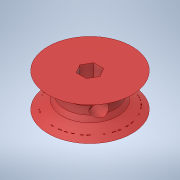
# Autodesk Inventor part: hexSpoolForArmV01
Saved by Autodesk Inventor 2022.2 (Build 262287010, 287A)
## iProperties
Created: 2019-02-24
Part Number: hexSpoolForArmV01
Material: PC/ABS Plastic
Document SubType Name: Modeling
Designer: steele
Density: 0.357273 g/cm^3
Appearance: Smooth - Red
holeForString: 0.200 in
stringDiameter: 0.120 in
clearanceForString: 0.080 in
clearanceForHexShaft: 0.020 in
spoolInteriorDiameter: 1.500 in
spoolInteriroRadius: 0.750 in
spoolExteriorDiameter: 2.500 in
spoolExteriorRadius: 1.250 in
hexHoleChamfer: 0.063 in
stringHoleCenterFromHexShaft: 0.360 in
textCircleDiameter: 1.875 in
textHeight: 0.180 in
textDepth: 0.050 in
Author: steele
Autodesk Inventor part; units mm, degrees
(part 1 of 2)
ref_plane "XZ Plane" through (0, 0, 0) normal (0, 1, 0) x (-1, 0, 0)
ref_plane "XY Plane" through (0, 0, 0) normal (0, 0, 1) x (1, 0, 0)
sketch "Sketch15" plane through (0, 0, 0) normal (0, 0, 1) x (1, 0, 0)
  line L0 (31.75, 0) -> (31.75, 50.8) construction
  line L1 (12.065, 0) -> (31.75, 0)
  line L2 (19.05, 0) -> (19.05, 50.8) construction
  line L3 (0, 50.8) -> (0, 0)
  line L4 (19.05, 12.7) -> (31.75, 12.7) construction
  line L5 (31.75, 0) -> (19.05, 7.3323)
  line L6 (31.75, 25.4) -> (19.05, 18.0677)
  line L7 (19.05, 18.0677) -> (31.75, 18.0677) construction
  line L8 (19.05, 18.0677) -> (19.05, 7.3323)
  line L9 (31.75, 25.4) -> (19.05, 32.7323)
  line L10 (19.05, 32.7323) -> (19.05, 43.4677)
  line L11 (19.05, 43.4677) -> (31.75, 50.8)
  line L12 (31.75, 25.4) -> (19.05, 25.4) construction
  line L13 (19.05, 43.4677) -> (31.75, 43.4677) construction
  line L14 (12.065, 0) -> (0, 0)
  line L15 (31.75, 50.8) -> (0, 50.8)
  dimension "d86" = 50.8
  dimension "d89" = 25.4
  dimension "centerLineForSpool" = 12.7
  dimension "d93" = 30
  dimension "d94" = 30
  dimension "d95" = 30
  dimension "d96" = 30
  dimension "d156" = 31.75
  dimension "d158" = 31.75
  constraints: 32 end point, 9 point on line, 3 horizontal, 2 midpoint, 2 perpendicular, 1 collinear, 1 vertical
  measures "d86" distance of L0.start L0.end
  measures "d89" distance from line of L6.start L1
  measures "centerLineForSpool" distance from line of L4.start L1
  measures "d93" angle of L5 L1
  measures "d94" angle of L6 L7
  measures "d95" angle of L9 L12
  measures "d96" angle of L11 L13
  measures "d156" distance from line of L0.end L3
  measures "d158" distance from line of L0.start L3
revolve "Revolution2" add sketch "Sketch15" angle 360 about axis through (0, 50.8, 0) along (0, -1, 0)
sketch "Sketch16" plane through (0, 0, 0) normal (0, -1, 0) x (1, 0, 0)
  line L0 (-7.6256, 0) -> (-3.8128, 6.604)
  line L1 (-3.8128, 6.604) -> (3.8128, 6.604)
  line L2 (3.8128, 6.604) -> (7.6256, 0)
  line L3 (7.6256, 0) -> (3.8128, -6.604)
  line L4 (3.8128, -6.604) -> (-3.8128, -6.604)
  line L5 (-3.8128, -6.604) -> (-7.6256, 0)
  point P0 (0, 0)
  point P1 (0, 0)
  dimension "d103" = 13.208
  constraints: 12 end point, 1 coincident, 1 horizontal, 13 other
  measures "d103" distance between parallel lines of L1 L4
extrude "Extrusion11" cut sketch "Sketch16" against normal through all
sketch "Sketch17" plane through (0, 0, 0) normal (1, 0, 0) x (0, 1, 0)
  circle A0 centre (38.1, 9.144) radius 2.54
  circle A1 centre (12.7, 9.144) radius 2.54
  line L0 (0, 31.75) -> (0, -31.75) projected
  line L1 (50.8, 31.75) -> (50.8, -31.75) projected
  line L2 (0, 6.604) -> (50.8, 6.604) projected
  point P0 (0, 0)
  point P1 (50.8, -31.75)
  point P2 (69.85, 6.858)
  point P3 (72.39, 6.858)
  point P4 (50.8, 6.604)
  dimension "d110" = 12.7
  dimension "d111" = 12.7
  dimension "d112" = 5.08
  constraints: 2 centre point, 1 equal radius, 4 other
  measures "d110" distance from line of A1.centre L0
  measures "d112" diameter of A0
extrude "Extrusion13" cut sketch "Sketch17" along normal through all both and the other way through all
ref_plane "Work Plane4" through (-19.05, 0, 0) normal (1, 0, 0) x (0, 1, 0)
sketch "Sketch22" plane through (-19.05, 0, 0) normal (1, 0, 0) x (0, 1, 0)
  spline S0 degree 8 poles (40.64, 9.144) (40.64, 9.42) (40.6057, 9.6896) (40.54, 9.9488) (40.4456, 10.1945) (40.3253, 10.4241) (40.1822, 10.6353) (40.019, 10.8263) (39.6643, 11.1594) (39.4723, 11.3044) (39.2651, 11.4282) (39.0456, 11.5293) (38.8165, 11.6061) (38.5806, 11.6579) (38.3408, 11.684) (37.8188, 11.684) (37.5395, 11.6484) (37.2666, 11.5781) (37.0042, 11.4743) (36.7566, 11.3384) (36.5278, 11.1726) (36.322, 10.9796) (35.9648, 10.5477) (35.8095, 10.305) (35.6834, 10.0377) (35.5915, 9.75) (35.5382, 9.4472) (35.5271, 9.1354) (35.5605, 8.8213) (35.7533, 8.0702) (35.9537, 7.6667) (36.2256, 7.316) (36.5542, 7.0287) (36.9234, 6.8124) (37.3159, 6.6712) (37.7136, 6.604) (38.3775, 6.604) (38.6564, 6.6386) (38.9325, 6.7085) (39.2015, 6.8141) (39.4588, 6.9552) (39.6993, 7.1318) (39.9175, 7.3429) (40.2331, 7.7498) (40.3461, 7.9265) (40.4431, 8.1154) (40.522, 8.3139) (40.5815, 8.5192) (40.6208, 8.7281) (40.64, 8.9374) (40.64, 9.144) knots 0 0 0 0 0 0 0 0 0 0.12897 0.12897 0.12897 0.12897 0.12897 0.12897 0.12897 0.253758 0.253758 0.253758 0.253758 0.253758 0.253758 0.253758 0.399502 0.399502 0.399502 0.399502 0.399502 0.399502 0.399502 0.544455 0.544455 0.544455 0.544455 0.544455 0.544455 0.544455 0.751871 0.751871 0.751871 0.751871 0.751871 0.751871 0.751871 0.90085 0.90085 0.90085 0.90085 0.90085 0.90085 0.90085 1 1 1 1 1 1 1 1 1 projected
  circle A0 centre (38.1, 9.144) radius 4.7625
  circle A1 centre (38.1, 9.144) radius 2.54 construction
  line L0 (38.1, 6.604) -> (12.7, 6.604) construction
  line L1 (50.8, 31.75) -> (50.8, -31.75) construction
  point P0 (0, 0)
  point P1 (69.85, 6.858)
  point P2 (50.8, -31.75)
  point P3 (72.39, 6.858)
  point P4 (12.7, 6.604)
  dimension "d121" = 12.7
  dimension "d122" = 5.08
  dimension "d125" = 9.525
  constraints: 2 centre point, 1 concentric, 1 vertical alignment, 3 other
  measures "d122" diameter of A1
  measures "d125" diameter of A0
extrude "Extrusion16" cut sketch "Sketch22" along normal blind 11.1125
ref_plane "Work Plane5" through (19.05, 0, 0) normal (1, 0, 0) x (0, 1, 0)
sketch "Sketch23" plane through (19.05, 0, 0) normal (1, 0, 0) x (0, 1, 0)
  line L0 (12.7, 6.604) -> (38.1, 6.604) projected
  circle A0 centre (12.7, 9.144) radius 2.54 construction
  line L1 (0, 31.75) -> (0, -31.75) projected
  circle A1 centre (12.7, 9.144) radius 4.7625
  point P0 (0, 0)
  dimension "d127" = 5.08
  dimension "d128" = 12.7
  dimension "d129" = 9.525
  constraints: 2 centre point, 1 coincident, 1 tangent
  measures "d127" diameter of A0
  measures "d128" distance from line of A0.centre L1
  measures "d129" diameter of A1
extrude "Extrusion17" cut sketch "Sketch23" against normal blind 11.1125
chamfer "Chamfer12" distance 2.3813 angle 45 4 edges at (-19.05, 43.4677, 0) (-19.05, 32.7323, 0) (-19.05, 18.0677, 0) (-19.05, 7.3323, 0)
ref_plane "Work Plane6" through (0, 25.4, 0) normal (0, -1, 0) x (1, 0, 0)
sketch "Sketch26" plane through (0, 0, 0) normal (0, -1, 0) x (1, 0, 0)
  circle A0 centre (0, 0) radius 23.8125 construction
  spline S0 degree 2 poles (-24.7852, 3.5176) (-24.5019, 3.4962) (-24.0902, 3.2484) (-23.9621, 3.0591) knots 0 0 0 1 2 2 2
  spline S1 degree 2 poles (-23.9621, 3.0591) (-23.809, 2.8308) (-23.706, 2.3091) (-23.7359, 1.9119) knots 0 0 0 1 2 2 2
  line L0 (-23.7359, 1.9119) -> (-23.8505, 0.3941)
  line L1 (-23.8505, 0.3941) -> (-27.6497, 0.6808)
  line L2 (-27.6497, 0.6808) -> (-27.5486, 2.02)
  spline S2 degree 2 poles (-27.5486, 2.02) (-27.517, 2.4388) (-27.4198, 2.8649) (-27.3041, 3.045) knots 0 0 0 1 2 2 2
  spline S3 degree 2 poles (-27.3041, 3.045) (-27.1807, 3.2432) (-26.7962, 3.4154) (-26.556, 3.3973) knots 0 0 0 1 2 2 2
  spline S4 degree 2 poles (-26.556, 3.3973) (-26.2789, 3.3764) (-25.8657, 3.0665) (-25.7827, 2.8126) knots 0 0 0 1 2 2 2
  line L3 (-25.7827, 2.8126) -> (-25.7643, 2.8112)
  spline S5 degree 2 poles (-25.7643, 2.8112) (-25.6637, 3.1597) (-25.1731, 3.5468) (-24.7852, 3.5176) knots 0 0 0 1 2 2 2
  spline S6 degree 2 poles (-24.8749, 2.5335) (-25.0535, 2.547) (-25.2643, 2.4205) (-25.3273, 2.2828) knots 0 0 0 1 2 2 2
  spline S7 degree 2 poles (-25.3273, 2.2828) (-25.3677, 2.1992) (-25.3968, 1.8948) (-25.4159, 1.6424) knots 0 0 0 1 2 2 2
  line L4 (-25.4159, 1.6424) -> (-25.4291, 1.4669)
  line L5 (-25.4291, 1.4669) -> (-24.4716, 1.3946)
  line L6 (-24.4716, 1.3946) -> (-24.4677, 1.447)
  spline S8 degree 2 poles (-24.4677, 1.447) (-24.4398, 1.8164) (-24.4277, 2.1004) (-24.4812, 2.253) knots 0 0 0 1 2 2 2
  spline S9 degree 2 poles (-24.4812, 2.253) (-24.5299, 2.3867) (-24.7364, 2.5231) (-24.8749, 2.5335) knots 0 0 0 1 2 2 2
  spline S10 degree 2 poles (-26.4414, 2.4133) (-26.5338, 2.4203) (-26.7349, 2.3395) (-26.7855, 2.2442) knots 0 0 0 1 2 2 2
  spline S11 degree 2 poles (-26.7855, 2.2442) (-26.8355, 2.1551) (-26.8612, 1.897) (-26.8805, 1.6414) knots 0 0 0 1 2 2 2
  line L7 (-26.8805, 1.6414) -> (-26.8854, 1.5768)
  line L8 (-26.8854, 1.5768) -> (-26.0787, 1.5159)
  line L9 (-26.0787, 1.5159) -> (-26.0697, 1.636)
  spline S12 degree 2 poles (-26.0697, 1.636) (-26.0513, 1.8792) (-26.0457, 2.0769) (-26.0871, 2.1853) knots 0 0 0 1 2 2 2
  spline S13 degree 2 poles (-26.0871, 2.1853) (-26.1339, 2.3034) (-26.3152, 2.4038) (-26.4414, 2.4133) knots 0 0 0 1 2 2 2
  spline S14 degree 2 poles (-24.3269, 6.9191) (-23.6337, 6.7652) (-23.0058, 5.832) (-23.159, 5.1418) knots 0 0 0 1 2 2 2
  spline S15 degree 2 poles (-23.159, 5.1418) (-23.3116, 4.4545) (-24.2766, 3.8686) (-24.9698, 4.0224) knots 0 0 0 1 2 2 2
  spline S16 degree 2 poles (-24.9698, 4.0224) (-25.6691, 4.1776) (-26.2926, 5.1162) (-26.1401, 5.8034) knots 0 0 0 1 2 2 2
  spline S17 degree 2 poles (-26.1401, 5.8034) (-25.9875, 6.4906) (-25.0232, 7.0736) (-24.3269, 6.9191) knots 0 0 0 1 2 2 2
  spline S18 degree 2 poles (-24.5196, 6.0225) (-24.7698, 6.078) (-25.1224, 6.0709) (-25.2379, 6.0207) knots 0 0 0 1 2 2 2
  spline S19 degree 2 poles (-25.2379, 6.0207) (-25.3608, 5.9657) (-25.4857, 5.7878) (-25.5131, 5.6643) knots 0 0 0 1 2 2 2
  spline S20 degree 2 poles (-25.5131, 5.6643) (-25.5399, 5.5437) (-25.5097, 5.3377) (-25.4246, 5.2366) knots 0 0 0 1 2 2 2
  spline S21 degree 2 poles (-25.4246, 5.2366) (-25.3449, 5.1399) (-25.0243, 4.9738) (-24.7651, 4.9163) knots 0 0 0 1 2 2 2
  spline S22 degree 2 poles (-24.7651, 4.9163) (-24.5089, 4.8594) (-24.1737, 4.8736) (-24.0618, 4.9215) knots 0 0 0 1 2 2 2
  spline S23 degree 2 poles (-24.0618, 4.9215) (-23.95, 4.9694) (-23.8127, 5.1604) (-23.7846, 5.287) knots 0 0 0 1 2 2 2
  spline S24 degree 2 poles (-23.7846, 5.287) (-23.7612, 5.3924) (-23.8035, 5.6295) (-23.8792, 5.7159) knots 0 0 0 1 2 2 2
  spline S25 degree 2 poles (-23.8792, 5.7159) (-23.968, 5.8147) (-24.2543, 5.9636) (-24.5196, 6.0225) knots 0 0 0 1 2 2 2
  spline S26 degree 2 poles (-22.3455, 8.0742) (-22.5236, 7.5576) (-23.1127, 7.2315) (-23.5973, 7.3985) knots 0 0 0 1 2 2 2
  line L10 (-23.5973, 7.3985) -> (-24.8671, 7.8361)
  line L11 (-24.8671, 7.8361) -> (-24.9787, 7.5121)
  line L12 (-24.9787, 7.5121) -> (-25.5684, 7.7153)
  line L13 (-25.5684, 7.7153) -> (-25.4567, 8.0393)
  line L14 (-25.4567, 8.0393) -> (-26.2332, 8.3069)
  line L15 (-26.2332, 8.3069) -> (-25.9415, 9.1534)
  line L16 (-25.9415, 9.1534) -> (-25.165, 8.8858)
  line L17 (-25.165, 8.8858) -> (-24.8834, 9.7031)
  line L18 (-24.8834, 9.7031) -> (-24.2937, 9.4999)
  line L19 (-24.2937, 9.4999) -> (-24.5754, 8.6826)
  line L20 (-24.5754, 8.6826) -> (-23.6092, 8.3497)
  spline S27 degree 2 poles (-23.6092, 8.3497) (-23.4661, 8.3004) (-23.251, 8.2328) (-23.1543, 8.2386) knots 0 0 0 1 2 2 2
  spline S28 degree 2 poles (-23.1543, 8.2386) (-23.0576, 8.2445) (-22.899, 8.3825) (-22.8426, 8.546) knots 0 0 0 1 2 2 2
  spline S29 degree 2 poles (-22.8426, 8.546) (-22.8185, 8.616) (-22.8014, 8.8551) (-22.8097, 8.9069) knots 0 0 0 1 2 2 2
  line L21 (-22.8097, 8.9069) -> (-22.7846, 8.9799)
  line L22 (-22.7846, 8.9799) -> (-22.1891, 8.7747)
  spline S30 degree 2 poles (-22.1891, 8.7747) (-22.2013, 8.6254) (-22.2671, 8.3019) (-22.3455, 8.0742) knots 0 0 0 1 2 2 2
  spline S31 degree 2 poles (-21.5159, 10.0789) (-21.7403, 9.5806) (-22.3567, 9.3097) (-22.824, 9.5202) knots 0 0 0 1 2 2 2
  line L23 (-22.824, 9.5202) -> (-24.0486, 10.0718)
  line L24 (-24.0486, 10.0718) -> (-24.1894, 9.7593)
  line L25 (-24.1894, 9.7593) -> (-24.758, 10.0154)
  line L26 (-24.758, 10.0154) -> (-24.6173, 10.3279)
  line L27 (-24.6173, 10.3279) -> (-25.3661, 10.6652)
  line L28 (-25.3661, 10.6652) -> (-24.9984, 11.4816)
  line L29 (-24.9984, 11.4816) -> (-24.2495, 11.1443)
  line L30 (-24.2495, 11.1443) -> (-23.8945, 11.9325)
  line L31 (-23.8945, 11.9325) -> (-23.3259, 11.6764)
  line L32 (-23.3259, 11.6764) -> (-23.6809, 10.8882)
  line L33 (-23.6809, 10.8882) -> (-22.7491, 10.4685)
  spline S32 degree 2 poles (-22.7491, 10.4685) (-22.6111, 10.4063) (-22.4031, 10.3194) (-22.3062, 10.3164) knots 0 0 0 1 2 2 2
  spline S33 degree 2 poles (-22.3062, 10.3164) (-22.2094, 10.3134) (-22.0389, 10.4364) (-21.9679, 10.594) knots 0 0 0 1 2 2 2
  spline S34 degree 2 poles (-21.9679, 10.594) (-21.9374, 10.6616) (-21.8986, 10.8981) (-21.9021, 10.9505) knots 0 0 0 1 2 2 2
  line L34 (-21.9021, 10.9505) -> (-21.8704, 11.0208)
  line L35 (-21.8704, 11.0208) -> (-21.2961, 10.7622)
  spline S35 degree 2 poles (-21.2961, 10.7622) (-21.322, 10.6147) (-21.4169, 10.2985) (-21.5159, 10.0789) knots 0 0 0 1 2 2 2
  spline S36 degree 2 poles (-20.9405, 14.1834) (-20.3302, 13.8203) (-20.0259, 12.7376) (-20.3873, 12.1299) knots 0 0 0 1 2 2 2
  spline S37 degree 2 poles (-20.3873, 12.1299) (-20.7473, 11.5249) (-21.8471, 11.2703) (-22.4574, 11.6334) knots 0 0 0 1 2 2 2
  spline S38 degree 2 poles (-22.4574, 11.6334) (-23.0731, 11.9996) (-23.3716, 13.0861) (-23.0117, 13.6911) knots 0 0 0 1 2 2 2
  spline S39 degree 2 poles (-23.0117, 13.6911) (-22.6518, 14.2961) (-21.5534, 14.548) (-20.9405, 14.1834) knots 0 0 0 1 2 2 2
  spline S40 degree 2 poles (-21.404, 13.3921) (-21.6242, 13.5232) (-21.9614, 13.6267) (-22.0868, 13.6151) knots 0 0 0 1 2 2 2
  spline S41 degree 2 poles (-22.0868, 13.6151) (-22.2208, 13.6014) (-22.395, 13.4715) (-22.4597, 13.3627) knots 0 0 0 1 2 2 2
  spline S42 degree 2 poles (-22.4597, 13.3627) (-22.5229, 13.2566) (-22.5586, 13.0516) (-22.5095, 12.9289) knots 0 0 0 1 2 2 2
  spline S43 degree 2 poles (-22.5095, 12.9289) (-22.464, 12.812) (-22.2115, 12.5541) (-21.9833, 12.4183) knots 0 0 0 1 2 2 2
  spline S44 degree 2 poles (-21.9833, 12.4183) (-21.7578, 12.2841) (-21.435, 12.1927) (-21.3137, 12.2032) knots 0 0 0 1 2 2 2
  spline S45 degree 2 poles (-21.3137, 12.2032) (-21.1925, 12.2137) (-21.0024, 12.3521) (-20.9361, 12.4636) knots 0 0 0 1 2 2 2
  spline S46 degree 2 poles (-20.9361, 12.4636) (-20.8809, 12.5564) (-20.8468, 12.7948) (-20.8917, 12.9006) knots 0 0 0 1 2 2 2
  spline S47 degree 2 poles (-20.8917, 12.9006) (-20.9451, 13.0222) (-21.1705, 13.2532) (-21.404, 13.3921) knots 0 0 0 1 2 2 2
  line L36 (-17.2449, 16.4705) -> (-18.3346, 17.4051)
  spline S48 degree 2 poles (-18.3346, 17.4051) (-18.4963, 17.5438) (-18.7267, 17.7211) (-18.8211, 17.7532) knots 0 0 0 1 2 2 2
  spline S49 degree 2 poles (-18.8211, 17.7532) (-18.9176, 17.7831) (-19.0854, 17.7155) (-19.1798, 17.6053) knots 0 0 0 1 2 2 2
  spline S50 degree 2 poles (-19.1798, 17.6053) (-19.2462, 17.528) (-19.3068, 17.3197) (-19.3199, 17.1764) knots 0 0 0 1 2 2 2
  line L37 (-19.3199, 17.1764) -> (-17.7755, 15.8518)
  line L38 (-17.7755, 15.8518) -> (-18.3624, 15.1674)
  line L39 (-18.3624, 15.1674) -> (-19.4522, 16.1021)
  spline S51 degree 2 poles (-19.4522, 16.1021) (-19.6116, 16.2388) (-19.8463, 16.4157) (-19.9407, 16.4479) knots 0 0 0 1 2 2 2
  spline S52 degree 2 poles (-19.9407, 16.4479) (-20.0372, 16.4777) (-20.205, 16.4101) (-20.2994, 16.2999) knots 0 0 0 1 2 2 2
  spline S53 degree 2 poles (-20.2994, 16.2999) (-20.3698, 16.2179) (-20.4311, 15.9899) (-20.4416, 15.8686) knots 0 0 0 1 2 2 2
  line L40 (-20.4416, 15.8686) -> (-18.8971, 14.544)
  line L41 (-18.8971, 14.544) -> (-19.48, 13.8644)
  line L42 (-19.48, 13.8644) -> (-21.6619, 15.7357)
  line L43 (-21.6619, 15.7357) -> (-21.079, 16.4154)
  line L44 (-21.079, 16.4154) -> (-20.8376, 16.2083)
  spline S54 degree 2 poles (-20.8376, 16.2083) (-20.8355, 16.4953) (-20.7396, 16.9297) (-20.5808, 17.1148) knots 0 0 0 1 2 2 2
  spline S55 degree 2 poles (-20.5808, 17.1148) (-20.41, 17.314) (-19.9588, 17.4559) (-19.7007, 17.3727) knots 0 0 0 1 2 2 2
  spline S56 degree 2 poles (-19.7007, 17.3727) (-19.7166, 17.724) (-19.616, 18.2397) (-19.4632, 18.4179) knots 0 0 0 1 2 2 2
  spline S57 degree 2 poles (-19.4632, 18.4179) (-19.3326, 18.5702) (-19.0294, 18.7292) (-18.8607, 18.7268) knots 0 0 0 1 2 2 2
  spline S58 degree 2 poles (-18.8607, 18.7268) (-18.6768, 18.7277) (-18.3102, 18.5719) (-18.0781, 18.3729) knots 0 0 0 1 2 2 2
  line L45 (-18.0781, 18.3729) -> (-16.6579, 17.1548)
  line L46 (-16.6579, 17.1548) -> (-17.2449, 16.4705)
  line L47 (-12.3046, 20.4503) -> (-13.0897, 19.9027)
  line L48 (-13.0897, 19.9027) -> (-14.0558, 21.2879)
  line L49 (-14.0558, 21.2879) -> (-15.122, 20.5443)
  line L50 (-15.122, 20.5443) -> (-14.1558, 19.1591)
  line L51 (-14.1558, 19.1591) -> (-14.9408, 18.6115)
  line L52 (-14.9408, 18.6115) -> (-17.1205, 21.7365)
  line L53 (-17.1205, 21.7365) -> (-16.3354, 22.284)
  line L54 (-16.3354, 22.284) -> (-15.537, 21.1394)
  line L55 (-15.537, 21.1394) -> (-14.4709, 21.883)
  line L56 (-14.4709, 21.883) -> (-15.2693, 23.0277)
  line L57 (-15.2693, 23.0277) -> (-14.4843, 23.5752)
  line L58 (-14.4843, 23.5752) -> (-12.3046, 20.4503)
  spline S59 degree 2 poles (-10.3027, 21.3842) (-11.0331, 21.0225) (-12.1559, 21.3346) (-12.4752, 21.9792) knots 0 0 0 1 2 2 2
  spline S60 degree 2 poles (-12.4752, 21.9792) (-12.7877, 22.61) (-12.4356, 23.7216) (-11.7826, 24.0451) knots 0 0 0 1 2 2 2
  spline S61 degree 2 poles (-11.7826, 24.0451) (-11.1933, 24.337) (-10.2791, 23.9939) (-9.9859, 23.4018) knots 0 0 0 1 2 2 2
  line L59 (-9.9859, 23.4018) -> (-9.842, 23.1113)
  line L60 (-9.842, 23.1113) -> (-11.6044, 22.2383)
  spline S62 degree 2 poles (-11.6044, 22.2383) (-11.5042, 22.064) (-11.2563, 21.8904) (-11.1156, 21.8706) knots 0 0 0 1 2 2 2
  spline S63 degree 2 poles (-11.1156, 21.8706) (-10.9776, 21.8493) (-10.6708, 21.9255) (-10.5075, 22.0064) knots 0 0 0 1 2 2 2
  spline S64 degree 2 poles (-10.5075, 22.0064) (-10.3692, 22.0749) (-10.1282, 22.2701) (-10.0408, 22.3788) knots 0 0 0 1 2 2 2
  spline S65 degree 2 poles (-10.0408, 22.3788) (-9.9617, 22.4697) (-9.8464, 22.6542) (-9.8131, 22.719) knots 0 0 0 1 2 2 2
  line L61 (-9.8131, 22.719) -> (-9.7273, 22.7615)
  line L62 (-9.7273, 22.7615) -> (-9.3984, 22.0975)
  spline S66 degree 2 poles (-9.3984, 22.0975) (-9.4788, 22.0094) (-9.6064, 21.8635) (-9.7338, 21.7591) knots 0 0 0 1 2 2 2
  spline S67 degree 2 poles (-9.7338, 21.7591) (-9.846, 21.6587) (-10.1035, 21.4829) (-10.3027, 21.3842) knots 0 0 0 1 2 2 2
  spline S68 degree 2 poles (-10.8731, 23.2035) (-11.0047, 23.4553) (-11.3617, 23.6127) (-11.5914, 23.4989) knots 0 0 0 1 2 2 2
  spline S69 degree 2 poles (-11.5914, 23.4989) (-11.8265, 23.3824) (-11.9524, 22.9687) (-11.847, 22.7211) knots 0 0 0 1 2 2 2
  line L63 (-11.847, 22.7211) -> (-10.8731, 23.2035)
  line L64 (-6.1681, 23.0543) -> (-7.1619, 22.7162)
  line L65 (-7.1619, 22.7162) -> (-7.9447, 23.3207)
  line L66 (-7.9447, 23.3207) -> (-8.2113, 22.3593)
  line L67 (-8.2113, 22.3593) -> (-9.1847, 22.0283)
  line L68 (-9.1847, 22.0283) -> (-8.6453, 23.7314)
  line L69 (-8.6453, 23.7314) -> (-10.0927, 24.7556)
  line L70 (-10.0927, 24.7556) -> (-9.0989, 25.0936)
  line L71 (-9.0989, 25.0936) -> (-8.3298, 24.5008)
  line L72 (-8.3298, 24.5008) -> (-8.0787, 25.4406)
  line L73 (-8.0787, 25.4406) -> (-7.1053, 25.7717)
  line L74 (-7.1053, 25.7717) -> (-7.6351, 24.0979)
  line L75 (-7.6351, 24.0979) -> (-6.1681, 23.0543)
  line L76 (-4.7798, 23.3323) -> (-5.6624, 23.1339)
  line L77 (-5.6624, 23.1339) -> (-5.8832, 24.1159)
  line L78 (-5.8832, 24.1159) -> (-5.0006, 24.3143)
  line L79 (-5.0006, 24.3143) -> (-4.7798, 23.3323)
  line L80 (-5.1895, 25.1547) -> (-6.0721, 24.9563)
  line L81 (-6.0721, 24.9563) -> (-6.2929, 25.9383)
  line L82 (-6.2929, 25.9383) -> (-5.4103, 26.1368)
  line L83 (-5.4103, 26.1368) -> (-5.1895, 25.1547)
  spline S70 degree 2 poles (0.2628, 25.758) (0.2859, 25.2646) (0.1633, 24.517) (-0.0008, 24.259) knots 0 0 0 1 2 2 2
  spline S71 degree 2 poles (-0.0008, 24.259) (-0.1619, 24.0041) (-0.7083, 23.7251) (-1.1092, 23.7063) knots 0 0 0 1 2 2 2
  spline S72 degree 2 poles (-1.1092, 23.7063) (-1.5133, 23.6874) (-2.0803, 23.9142) (-2.2679, 24.1589) knots 0 0 0 1 2 2 2
  spline S73 degree 2 poles (-2.2679, 24.1589) (-2.4554, 24.4005) (-2.6471, 25.1271) (-2.6702, 25.6206) knots 0 0 0 1 2 2 2
  spline S74 degree 2 poles (-2.6702, 25.6206) (-2.6939, 26.1264) (-2.5701, 26.8493) (-2.4034, 27.1167) knots 0 0 0 1 2 2 2
  spline S75 degree 2 poles (-2.4034, 27.1167) (-2.2364, 27.378) (-1.6835, 27.6512) (-1.2949, 27.6694) knots 0 0 0 1 2 2 2
  spline S76 degree 2 poles (-1.2949, 27.6694) (-0.8848, 27.6886) (-0.3236, 27.4553) (-0.1358, 27.2075) knots 0 0 0 1 2 2 2
  spline S77 degree 2 poles (-0.1358, 27.2075) (0.0486, 26.9658) (0.2404, 26.2361) (0.2628, 25.758) knots 0 0 0 1 2 2 2
  spline S78 degree 2 poles (-0.6964, 25.7131) (-0.7295, 26.4194) (-0.9875, 26.9791) (-1.262, 26.9662) knots 0 0 0 1 2 2 2
  spline S79 degree 2 poles (-1.262, 26.9662) (-1.5365, 26.9534) (-1.7441, 26.3718) (-1.7109, 25.6625) knots 0 0 0 1 2 2 2
  spline S80 degree 2 poles (-1.7109, 25.6625) (-1.6782, 24.9654) (-1.4167, 24.3966) (-1.1422, 24.4095) knots 0 0 0 1 2 2 2
  spline S81 degree 2 poles (-1.1422, 24.4095) (-0.8708, 24.4222) (-0.6636, 25.013) (-0.6964, 25.7131) knots 0 0 0 1 2 2 2
  line L84 (1.8183, 23.7473) -> (0.9151, 23.7992)
  line L85 (0.9151, 23.7992) -> (0.973, 24.8041)
  line L86 (0.973, 24.8041) -> (1.8761, 24.7521)
  line L87 (1.8761, 24.7521) -> (1.8183, 23.7473)
  spline S82 degree 2 poles (5.4564, 24.5447) (5.4082, 24.2491) (5.1255, 23.7822) (4.8981, 23.6347) knots 0 0 0 1 2 2 2
  spline S83 degree 2 poles (4.8981, 23.6347) (4.6707, 23.4873) (4.096, 23.3777) (3.6998, 23.4424) knots 0 0 0 1 2 2 2
  spline S84 degree 2 poles (3.6998, 23.4424) (3.2798, 23.5141) (2.6988, 23.7497) (2.5152, 23.8704) knots 0 0 0 1 2 2 2
  line L88 (2.5152, 23.8704) -> (2.649, 24.6901)
  line L89 (2.649, 24.6901) -> (2.7343, 24.6761)
  spline S85 degree 2 poles (2.7343, 24.6761) (2.801, 24.6246) (2.9608, 24.4921) (3.0951, 24.4139) knots 0 0 0 1 2 2 2
  spline S86 degree 2 poles (3.0951, 24.4139) (3.2207, 24.3402) (3.4866, 24.2249) (3.6541, 24.1975) knots 0 0 0 1 2 2 2
  spline S87 degree 2 poles (3.6541, 24.1975) (3.8004, 24.1736) (4.1536, 24.1911) (4.2732, 24.2717) knots 0 0 0 1 2 2 2
  spline S88 degree 2 poles (4.2732, 24.2717) (4.3618, 24.3354) (4.4774, 24.5074) (4.5028, 24.6628) knots 0 0 0 1 2 2 2
  spline S89 degree 2 poles (4.5028, 24.6628) (4.5247, 24.7969) (4.4458, 25.0037) (4.3669, 25.076) knots 0 0 0 1 2 2 2
  spline S90 degree 2 poles (4.3669, 25.076) (4.2529, 25.1822) (3.8951, 25.2907) (3.7641, 25.312) knots 0 0 0 1 2 2 2
  spline S91 degree 2 poles (3.7641, 25.312) (3.5569, 25.3459) (3.1529, 25.343) (3.0037, 25.3298) knots 0 0 0 1 2 2 2
  line L90 (3.0037, 25.3298) -> (2.9214, 25.3432)
  line L91 (2.9214, 25.3432) -> (3.2661, 27.4549)
  line L92 (3.2661, 27.4549) -> (5.7587, 27.0481)
  line L93 (5.7587, 27.0481) -> (5.6428, 26.3381)
  line L94 (5.6428, 26.3381) -> (4.043, 26.5992)
  line L95 (4.043, 26.5992) -> (3.9411, 25.9745)
  spline S92 degree 2 poles (3.9411, 25.9745) (4.0183, 25.9682) (4.2295, 25.94) (4.2874, 25.9305) knots 0 0 0 1 2 2 2
  spline S93 degree 2 poles (4.2874, 25.9305) (4.5586, 25.8862) (4.9978, 25.7019) (5.1592, 25.5598) knots 0 0 0 1 2 2 2
  spline S94 degree 2 poles (5.1592, 25.5598) (5.3496, 25.3849) (5.5112, 24.8798) (5.4564, 24.5447) knots 0 0 0 1 2 2 2
  line L96 (8.5255, 22.2857) -> (5.8517, 23.1179)
  line L97 (5.8517, 23.1179) -> (6.0361, 23.7105)
  spline S95 degree 2 poles (6.0361, 23.7105) (6.4595, 23.8762) (7.1506, 24.1849) (7.421, 24.3368) knots 0 0 0 1 2 2 2
  spline S96 degree 2 poles (7.421, 24.3368) (7.7765, 24.5334) (8.1483, 24.8865) (8.218, 25.1106) knots 0 0 0 1 2 2 2
  spline S97 degree 2 poles (8.218, 25.1106) (8.2969, 25.3641) (8.0777, 25.7299) (7.8065, 25.8143) knots 0 0 0 1 2 2 2
  spline S98 degree 2 poles (7.8065, 25.8143) (7.6679, 25.8574) (7.3992, 25.8667) (7.2559, 25.8531) knots 0 0 0 1 2 2 2
  spline S99 degree 2 poles (7.2559, 25.8531) (7.1147, 25.8356) (6.9011, 25.7727) (6.8477, 25.757) knots 0 0 0 1 2 2 2
  line L98 (6.8477, 25.757) -> (6.7769, 25.779)
  line L99 (6.7769, 25.779) -> (7.0237, 26.572)
  spline S100 degree 2 poles (7.0237, 26.572) (7.2, 26.598) (7.9022, 26.5476) (8.2058, 26.4531) knots 0 0 0 1 2 2 2
  spline S101 degree 2 poles (8.2058, 26.4531) (8.8544, 26.2513) (9.3408, 25.4661) (9.1784, 24.9443) knots 0 0 0 1 2 2 2
  spline S102 degree 2 poles (9.1784, 24.9443) (9.0784, 24.6229) (8.582, 24.0984) (8.1211, 23.8538) knots 0 0 0 1 2 2 2
  spline S103 degree 2 poles (8.1211, 23.8538) (7.8321, 23.7044) (7.3109, 23.4948) (7.1975, 23.4525) knots 0 0 0 1 2 2 2
  line L100 (7.1975, 23.4525) -> (8.7393, 22.9726)
  line L101 (8.7393, 22.9726) -> (8.5255, 22.2857)
  spline S104 degree 2 poles (12.3202, 22.6221) (12.109, 22.1755) (11.6499, 21.5729) (11.3839, 21.422) knots 0 0 0 1 2 2 2
  spline S105 degree 2 poles (11.3839, 21.422) (11.122, 21.2726) (10.5086, 21.2826) (10.1457, 21.4542) knots 0 0 0 1 2 2 2
  spline S106 degree 2 poles (10.1457, 21.4542) (9.7801, 21.6271) (9.3859, 22.0935) (9.335, 22.3976) knots 0 0 0 1 2 2 2
  spline S107 degree 2 poles (9.335, 22.3976) (9.2828, 22.6989) (9.4546, 23.4306) (9.6657, 23.8772) knots 0 0 0 1 2 2 2
  spline S108 degree 2 poles (9.6657, 23.8772) (9.8822, 24.3349) (10.3307, 24.9152) (10.6034, 25.0731) knots 0 0 0 1 2 2 2
  spline S109 degree 2 poles (10.6034, 25.0731) (10.8736, 25.2254) (11.4899, 25.2072) (11.8416, 25.0409) knots 0 0 0 1 2 2 2
  spline S110 degree 2 poles (11.8416, 25.0409) (12.2129, 24.8654) (12.5988, 24.396) (12.6484, 24.0891) knots 0 0 0 1 2 2 2
  spline S111 degree 2 poles (12.6484, 24.0891) (12.6978, 23.7891) (12.5247, 23.0547) (12.3202, 22.6221) knots 0 0 0 1 2 2 2
  spline S112 degree 2 poles (11.4521, 23.0325) (11.7543, 23.6717) (11.7891, 24.2871) (11.5407, 24.4045) knots 0 0 0 1 2 2 2
  spline S113 degree 2 poles (11.5407, 24.4045) (11.2923, 24.522) (10.836, 24.1059) (10.5325, 23.4639) knots 0 0 0 1 2 2 2
  spline S114 degree 2 poles (10.5325, 23.4639) (10.2342, 22.8331) (10.1982, 22.2081) (10.4466, 22.0906) knots 0 0 0 1 2 2 2
  spline S115 degree 2 poles (10.4466, 22.0906) (10.6923, 21.9745) (11.1525, 22.3989) (11.4521, 23.0325) knots 0 0 0 1 2 2 2
  line L102 (14.8417, 18.6496) -> (13.1842, 19.8561)
  line L103 (13.1842, 19.8561) -> (13.5748, 20.3928)
  line L104 (13.5748, 20.3928) -> (14.0167, 20.0712)
  line L105 (14.0167, 20.0712) -> (15.4775, 22.0782)
  line L106 (15.4775, 22.0782) -> (15.0356, 22.3998)
  line L107 (15.0356, 22.3998) -> (15.4263, 22.9365)
  line L108 (15.4263, 22.9365) -> (17.0838, 21.7301)
  line L109 (17.0838, 21.7301) -> (16.6932, 21.1934)
  line L110 (16.6932, 21.1934) -> (16.2513, 21.515)
  line L111 (16.2513, 21.515) -> (14.7905, 19.5079)
  line L112 (14.7905, 19.5079) -> (15.2324, 19.1863)
  line L113 (15.2324, 19.1863) -> (14.8417, 18.6496)
  spline S116 degree 2 poles (19.1212, 17.2884) (18.7512, 16.9032) (17.8332, 16.6206) (17.421, 16.7041) knots 0 0 0 1 2 2 2
  spline S117 degree 2 poles (17.421, 16.7041) (17.0746, 16.7714) (16.4944, 17.1747) (16.2117, 17.4463) knots 0 0 0 1 2 2 2
  line L114 (16.2117, 17.4463) -> (15.3522, 18.272)
  line L115 (15.3522, 18.272) -> (17.9919, 21.0195)
  line L116 (17.9919, 21.0195) -> (18.8424, 20.2023)
  spline S118 degree 2 poles (18.8424, 20.2023) (19.1318, 19.9243) (19.5666, 19.3652) (19.6524, 19.0088) knots 0 0 0 1 2 2 2
  spline S119 degree 2 poles (19.6524, 19.0088) (19.7549, 18.5763) (19.5041, 17.6869) (19.1212, 17.2884) knots 0 0 0 1 2 2 2
  spline S120 degree 2 poles (18.4175, 17.9731) (18.6785, 18.2447) (18.8637, 18.8118) (18.777, 19.1048) knots 0 0 0 1 2 2 2
  spline S121 degree 2 poles (18.777, 19.1048) (18.7095, 19.3153) (18.4172, 19.6261) (18.2035, 19.8314) knots 0 0 0 1 2 2 2
  line L117 (18.2035, 19.8314) -> (18.1901, 19.8443)
  line L118 (18.1901, 19.8443) -> (16.5366, 18.1232)
  line L119 (16.5366, 18.1232) -> (16.5499, 18.1104)
  spline S122 degree 2 poles (16.5499, 18.1104) (16.7815, 17.8879) (17.1148, 17.5976) (17.3473, 17.5499) knots 0 0 0 1 2 2 2
  spline S123 degree 2 poles (17.3473, 17.5499) (17.6191, 17.4942) (18.1565, 17.7014) (18.4175, 17.9731) knots 0 0 0 1 2 2 2
  line L120 (18.7665, 14.6649) -> (18.196, 15.3669)
  line L121 (18.196, 15.3669) -> (18.9772, 16.0017)
  line L122 (18.9772, 16.0017) -> (19.5477, 15.2996)
  line L123 (19.5477, 15.2996) -> (18.7665, 14.6649)
  line L124 (20.2162, 15.8429) -> (19.6457, 16.5449)
  line L125 (19.6457, 16.5449) -> (20.4268, 17.1797)
  line L126 (20.4268, 17.1797) -> (20.9973, 16.4776)
  line L127 (20.9973, 16.4776) -> (20.2162, 15.8429)
  line L128 (21.4602, 10.4073) -> (20.236, 12.6058)
  line L129 (20.236, 12.6058) -> (20.816, 12.9287)
  line L130 (20.816, 12.9287) -> (21.2065, 12.2274)
  line L131 (21.2065, 12.2274) -> (22.968, 13.2082)
  line L132 (22.968, 13.2082) -> (22.5774, 13.9096)
  line L133 (22.5774, 13.9096) -> (23.1196, 14.2115)
  spline S124 degree 2 poles (23.1196, 14.2115) (23.2053, 14.0577) (23.4155, 13.7754) (23.5097, 13.7078) knots 0 0 0 1 2 2 2
  spline S125 degree 2 poles (23.5097, 13.7078) (23.6222, 13.6326) (23.869, 13.6145) (24.0099, 13.6789) knots 0 0 0 1 2 2 2
  line L134 (24.0099, 13.6789) -> (24.4155, 12.9505)
  line L135 (24.4155, 12.9505) -> (21.6586, 11.4154)
  line L136 (21.6586, 11.4154) -> (22.0402, 10.7302)
  line L137 (22.0402, 10.7302) -> (21.4602, 10.4073)
  line L138 (22.0748, 8.941) -> (21.7194, 9.7729)
  line L139 (21.7194, 9.7729) -> (22.645, 10.1684)
  line L140 (22.645, 10.1684) -> (23.0004, 9.3365)
  line L141 (23.0004, 9.3365) -> (22.0748, 8.941)
  spline S126 degree 2 poles (24.4081, 6.0379) (24.122, 5.9496) (23.578, 5.9949) (23.3448, 6.133) knots 0 0 0 1 2 2 2
  spline S127 degree 2 poles (23.3448, 6.133) (23.1115, 6.271) (22.7576, 6.7369) (22.6392, 7.1204) knots 0 0 0 1 2 2 2
  spline S128 degree 2 poles (22.6392, 7.1204) (22.5165, 7.5284) (22.4689, 8.1535) (22.4952, 8.3717) knots 0 0 0 1 2 2 2
  line L142 (22.4952, 8.3717) -> (23.2888, 8.6167)
  line L143 (23.2888, 8.6167) -> (23.3143, 8.5341)
  spline S129 degree 2 poles (23.3143, 8.5341) (23.2978, 8.4515) (23.2504, 8.2494) (23.2401, 8.0944) knots 0 0 0 1 2 2 2
  spline S130 degree 2 poles (23.2401, 8.0944) (23.23, 7.9491) (23.245, 7.6597) (23.2951, 7.4974) knots 0 0 0 1 2 2 2
  spline S131 degree 2 poles (23.2951, 7.4974) (23.3388, 7.3558) (23.5116, 7.0472) (23.637, 6.9761) knots 0 0 0 1 2 2 2
  spline S132 degree 2 poles (23.637, 6.9761) (23.7335, 6.9251) (23.939, 6.8981) (24.0895, 6.9445) knots 0 0 0 1 2 2 2
  spline S133 degree 2 poles (24.0895, 6.9445) (24.2193, 6.9846) (24.3694, 7.1473) (24.399, 7.2501) knots 0 0 0 1 2 2 2
  spline S134 degree 2 poles (24.399, 7.2501) (24.4434, 7.3995) (24.3813, 7.7681) (24.3421, 7.895) knots 0 0 0 1 2 2 2
  spline S135 degree 2 poles (24.3421, 7.895) (24.2802, 8.0956) (24.0978, 8.4561) (24.0196, 8.5838) knots 0 0 0 1 2 2 2
  line L144 (24.0196, 8.5838) -> (23.995, 8.6635)
  line L145 (23.995, 8.6635) -> (26.0394, 9.2947)
  line L146 (26.0394, 9.2947) -> (26.7844, 6.8815)
  line L147 (26.7844, 6.8815) -> (26.0971, 6.6692)
  line L148 (26.0971, 6.6692) -> (25.6189, 8.2181)
  line L149 (25.6189, 8.2181) -> (25.0141, 8.0313)
  spline S136 degree 2 poles (25.0141, 8.0313) (25.0428, 7.9594) (25.1115, 7.7577) (25.1288, 7.7016) knots 0 0 0 1 2 2 2
  spline S137 degree 2 poles (25.1288, 7.7016) (25.2099, 7.4391) (25.2403, 6.9638) (25.1849, 6.756) knots 0 0 0 1 2 2 2
  spline S138 degree 2 poles (25.1849, 6.756) (25.113, 6.5076) (24.7326, 6.1381) (24.4081, 6.0379) knots 0 0 0 1 2 2 2
  line L150 (27.5311, 3.9195) -> (26.0206, 3.808)
  line L151 (26.0206, 3.808) -> (25.9288, 4.3248)
  line L152 (25.9288, 4.3248) -> (27.3853, 4.7402)
  line L153 (27.3853, 4.7402) -> (27.5311, 3.9195)
  line L154 (27.3427, 4.9804) -> (25.8322, 4.869)
  line L155 (25.8322, 4.869) -> (25.7404, 5.3858)
  line L156 (25.7404, 5.3858) -> (27.197, 5.8012)
  line L157 (27.197, 5.8012) -> (27.3427, 4.9804)
  spline S139 degree 2 poles (25.6584, -2.5378) (24.7325, -2.5129) (23.7005, -1.4966) (23.7236, -0.6386) knots 0 0 0 1 2 2 2
  spline S140 degree 2 poles (23.7236, -0.6386) (23.7469, 0.2225) (24.8443, 1.1751) (25.7579, 1.1504) knots 0 0 0 1 2 2 2
  spline S141 degree 2 poles (25.7579, 1.1504) (26.6746, 1.1257) (27.716, 0.1154) (27.6927, -0.7457) knots 0 0 0 1 2 2 2
  spline S142 degree 2 poles (27.6927, -0.7457) (27.6696, -1.6037) (26.5812, -2.5627) (25.6584, -2.5378) knots 0 0 0 1 2 2 2
  spline S143 degree 2 poles (25.685, -1.5502) (26.0276, -1.5594) (26.5098, -1.4335) (26.6642, -1.3172) knots 0 0 0 1 2 2 2
  spline S144 degree 2 poles (26.6642, -1.3172) (26.8249, -1.201) (26.969, -0.8961) (26.9735, -0.7294) knots 0 0 0 1 2 2 2
  spline S145 degree 2 poles (26.9735, -0.7294) (26.9783, -0.5535) (26.8595, -0.263) (26.7026, -0.126) knots 0 0 0 1 2 2 2
  spline S146 degree 2 poles (26.7026, -0.126) (26.5576, -0.0047) (26.0708, 0.1536) (25.7313, 0.1628) knots 0 0 0 1 2 2 2
  spline S147 degree 2 poles (25.7313, 0.1628) (25.3794, 0.1723) (24.9127, 0.0459) (24.752, -0.0703) knots 0 0 0 1 2 2 2
  spline S148 degree 2 poles (24.752, -0.0703) (24.5914, -0.1864) (24.4472, -0.4944) (24.4427, -0.6611) knots 0 0 0 1 2 2 2
  spline S149 degree 2 poles (24.4427, -0.6611) (24.4381, -0.8309) (24.5747, -1.1496) (24.7259, -1.268) knots 0 0 0 1 2 2 2
  spline S150 degree 2 poles (24.7259, -1.268) (24.8892, -1.3959) (25.327, -1.5405) (25.685, -1.5502) knots 0 0 0 1 2 2 2
  spline S151 degree 2 poles (24.8787, -6.7497) (24.3547, -6.6464) (23.6209, -6.0266) (23.4684, -5.6346) knots 0 0 0 1 2 2 2
  spline S152 degree 2 poles (23.4684, -5.6346) (23.3379, -5.3068) (23.3638, -4.6007) (23.4397, -4.216) knots 0 0 0 1 2 2 2
  line L158 (23.4397, -4.216) -> (23.6702, -3.0467)
  line L159 (23.6702, -3.0467) -> (27.4082, -3.7836)
  line L160 (27.4082, -3.7836) -> (27.1801, -4.9407)
  spline S153 degree 2 poles (27.1801, -4.9407) (27.1025, -5.3345) (26.867, -6.0025) (26.6134, -6.2672) knots 0 0 0 1 2 2 2
  spline S154 degree 2 poles (26.6134, -6.2672) (26.3049, -6.5871) (25.421, -6.8566) (24.8787, -6.7497) knots 0 0 0 1 2 2 2
  spline S155 degree 2 poles (25.0747, -5.7876) (25.4442, -5.8605) (26.0215, -5.7099) (26.2213, -5.4787) knots 0 0 0 1 2 2 2
  spline S156 degree 2 poles (26.2213, -5.4787) (26.3619, -5.3081) (26.4655, -4.8943) (26.5228, -4.6035) knots 0 0 0 1 2 2 2
  line L161 (26.5228, -4.6035) -> (26.5264, -4.5853)
  line L162 (26.5264, -4.5853) -> (24.1848, -4.1237)
  line L163 (24.1848, -4.1237) -> (24.1812, -4.1419)
  spline S157 degree 2 poles (24.1812, -4.1419) (24.1191, -4.4569) (24.0549, -4.8943) (24.1403, -5.1157) knots 0 0 0 1 2 2 2
  spline S158 degree 2 poles (24.1403, -5.1157) (24.2403, -5.3745) (24.7051, -5.7148) (25.0747, -5.7876) knots 0 0 0 1 2 2 2
  line L164 (24.2539, -8.4521) -> (24.5365, -7.5927)
  line L165 (24.5365, -7.5927) -> (25.4927, -7.9071)
  line L166 (25.4927, -7.9071) -> (25.2101, -8.7665)
  line L167 (25.2101, -8.7665) -> (24.2539, -8.4521)
  line L168 (22.4794, -7.8687) -> (22.762, -7.0093)
  line L169 (22.762, -7.0093) -> (23.7182, -7.3237)
  line L170 (23.7182, -7.3237) -> (23.4356, -8.183)
  line L171 (23.4356, -8.183) -> (22.4794, -7.8687)
  line L172 (20.3521, -12.4356) -> (21.5407, -10.2177)
  line L173 (21.5407, -10.2177) -> (22.1257, -10.5312)
  line L174 (22.1257, -10.5312) -> (21.7466, -11.2388)
  line L175 (21.7466, -11.2388) -> (23.5236, -12.1911)
  line L176 (23.5236, -12.1911) -> (23.9028, -11.4836)
  line L177 (23.9028, -11.4836) -> (24.4498, -11.7767)
  spline S159 degree 2 poles (24.4498, -11.7767) (24.3667, -11.9318) (24.2427, -12.2612) (24.2367, -12.3771) knots 0 0 0 1 2 2 2
  spline S160 degree 2 poles (24.2367, -12.3771) (24.2342, -12.5124) (24.3524, -12.7298) (24.4826, -12.8136) knots 0 0 0 1 2 2 2
  line L178 (24.4826, -12.8136) -> (24.0888, -13.5484)
  line L179 (24.0888, -13.5484) -> (21.3076, -12.0579)
  line L180 (21.3076, -12.0579) -> (20.9372, -12.7492)
  line L181 (20.9372, -12.7492) -> (20.3521, -12.4356)
  line L182 (19.4503, -13.745) -> (19.9583, -12.9965)
  line L183 (19.9583, -12.9965) -> (20.7911, -13.5617)
  line L184 (20.7911, -13.5617) -> (20.2831, -14.3102)
  line L185 (20.2831, -14.3102) -> (19.4503, -13.745)
  spline S161 degree 2 poles (18.7138, -17.7013) (18.3362, -17.3829) (17.8712, -16.7848) (17.7935, -16.489) knots 0 0 0 1 2 2 2
  spline S162 degree 2 poles (17.7935, -16.489) (17.7161, -16.1976) (17.8828, -15.6072) (18.1416, -15.3004) knots 0 0 0 1 2 2 2
  spline S163 degree 2 poles (18.1416, -15.3004) (18.4023, -14.9912) (18.9542, -14.7295) (19.2612, -14.7582) knots 0 0 0 1 2 2 2
  spline S164 degree 2 poles (19.2612, -14.7582) (19.5658, -14.7849) (20.2291, -15.1382) (20.6067, -15.4567) knots 0 0 0 1 2 2 2
  spline S165 degree 2 poles (20.6067, -15.4567) (20.9938, -15.7831) (21.4399, -16.3652) (21.5227, -16.6693) knots 0 0 0 1 2 2 2
  spline S166 degree 2 poles (21.5227, -16.6693) (21.6008, -16.9694) (21.4254, -17.5606) (21.1746, -17.858) knots 0 0 0 1 2 2 2
  spline S167 degree 2 poles (21.1746, -17.858) (20.9099, -18.1719) (20.3573, -18.4249) (20.048, -18.3942) knots 0 0 0 1 2 2 2
  spline S168 degree 2 poles (20.048, -18.3942) (19.7453, -18.3652) (19.0797, -18.0098) (18.7138, -17.7013) knots 0 0 0 1 2 2 2
  spline S169 degree 2 poles (19.3329, -16.9673) (19.8734, -17.4231) (20.4593, -17.6143) (20.6365, -17.4042) knots 0 0 0 1 2 2 2
  spline S170 degree 2 poles (20.6365, -17.4042) (20.8136, -17.1941) (20.5282, -16.6465) (19.9853, -16.1887) knots 0 0 0 1 2 2 2
  spline S171 degree 2 poles (19.9853, -16.1887) (19.4519, -15.7389) (18.8569, -15.5441) (18.6798, -15.7542) knots 0 0 0 1 2 2 2
  spline S172 degree 2 poles (18.6798, -15.7542) (18.5046, -15.9619) (18.7971, -16.5155) (19.3329, -16.9673) knots 0 0 0 1 2 2 2
  line L186 (18.9636, -20.3177) -> (18.0538, -19.1068)
  line L187 (18.0538, -19.1068) -> (18.4391, -18.7504)
  line L188 (18.4391, -18.7504) -> (19.5756, -19.7516)
  line L189 (19.5756, -19.7516) -> (18.9636, -20.3177)
  line L190 (18.1726, -21.0494) -> (17.2628, -19.8386)
  line L191 (17.2628, -19.8386) -> (17.6481, -19.4821)
  line L192 (17.6481, -19.4821) -> (18.7846, -20.4833)
  line L193 (18.7846, -20.4833) -> (18.1726, -21.0494)
  line L194 (10.9586, -21.202) -> (11.7773, -20.7063)
  line L195 (11.7773, -20.7063) -> (12.6521, -22.151)
  line L196 (12.6521, -22.151) -> (13.764, -21.4778)
  line L197 (13.764, -21.4778) -> (12.8893, -20.0331)
  line L198 (12.8893, -20.0331) -> (13.708, -19.5374)
  line L199 (13.708, -19.5374) -> (15.6813, -22.7965)
  line L200 (15.6813, -22.7965) -> (14.8626, -23.2922)
  line L201 (14.8626, -23.2922) -> (14.1398, -22.0984)
  line L202 (14.1398, -22.0984) -> (13.0279, -22.7717)
  line L203 (13.0279, -22.7717) -> (13.7507, -23.9655)
  line L204 (13.7507, -23.9655) -> (12.9319, -24.4612)
  line L205 (12.9319, -24.4612) -> (10.9586, -21.202)
  spline S173 degree 2 poles (9.2523, -21.8841) (9.7524, -21.6638) (10.3919, -21.8747) (10.5984, -22.3438) knots 0 0 0 1 2 2 2
  line L206 (10.5984, -22.3438) -> (11.1398, -23.5729)
  line L207 (11.1398, -23.5729) -> (11.4534, -23.4347)
  line L208 (11.4534, -23.4347) -> (11.7048, -24.0055)
  line L209 (11.7048, -24.0055) -> (11.3912, -24.1437)
  line L210 (11.3912, -24.1437) -> (11.7222, -24.8953)
  line L211 (11.7222, -24.8953) -> (10.9028, -25.2562)
  line L212 (10.9028, -25.2562) -> (10.5718, -24.5046)
  line L213 (10.5718, -24.5046) -> (9.7806, -24.853)
  line L214 (9.7806, -24.853) -> (9.5292, -24.2823)
  line L215 (9.5292, -24.2823) -> (10.3204, -23.9338)
  line L216 (10.3204, -23.9338) -> (9.9084, -22.9985)
  spline S174 degree 2 poles (9.9084, -22.9985) (9.8475, -22.8601) (9.751, -22.6563) (9.681, -22.5893) knots 0 0 0 1 2 2 2
  spline S175 degree 2 poles (9.681, -22.5893) (9.611, -22.5223) (9.4019, -22.4996) (9.2437, -22.5693) knots 0 0 0 1 2 2 2
  spline S176 degree 2 poles (9.2437, -22.5693) (9.1759, -22.5992) (8.9889, -22.749) (8.9564, -22.7903) knots 0 0 0 1 2 2 2
  line L217 (8.9564, -22.7903) -> (8.8858, -22.8214)
  line L218 (8.8858, -22.8214) -> (8.6319, -22.245)
  spline S177 degree 2 poles (8.6319, -22.245) (8.7498, -22.1526) (9.0319, -21.9811) (9.2523, -21.8841) knots 0 0 0 1 2 2 2
  line L219 (7.8748, -24.4475) -> (8.7308, -24.155)
  line L220 (8.7308, -24.155) -> (9.0563, -25.1074)
  line L221 (9.0563, -25.1074) -> (8.2002, -25.3999)
  line L222 (8.2002, -25.3999) -> (7.8748, -24.4475)
  line L223 (7.2707, -22.6799) -> (8.1268, -22.3874)
  line L224 (8.1268, -22.3874) -> (8.4522, -23.3398)
  line L225 (8.4522, -23.3398) -> (7.5962, -23.6324)
  line L226 (7.5962, -23.6324) -> (7.2707, -22.6799)
  spline S178 degree 2 poles (2.4494, -24.8874) (2.406, -24.6098) (2.5394, -24.1234) (2.7129, -23.9338) knots 0 0 0 1 2 2 2
  spline S179 degree 2 poles (2.7129, -23.9338) (2.8864, -23.7442) (3.3996, -23.489) (3.787, -23.4285) knots 0 0 0 1 2 2 2
  spline S180 degree 2 poles (3.787, -23.4285) (4.2263, -23.3598) (4.8776, -23.4081) (5.0902, -23.4686) knots 0 0 0 1 2 2 2
  line L227 (5.0902, -23.4686) -> (5.2179, -24.2861)
  line L228 (5.2179, -24.2861) -> (5.1264, -24.3004)
  spline S181 degree 2 poles (5.1264, -24.3004) (4.8985, -24.2017) (4.3097, -24.0937) (4.0779, -24.1299) knots 0 0 0 1 2 2 2
  spline S182 degree 2 poles (4.0779, -24.1299) (3.9406, -24.1513) (3.6279, -24.2502) (3.5305, -24.3467) knots 0 0 0 1 2 2 2
  spline S183 degree 2 poles (3.5305, -24.3467) (3.4551, -24.4241) (3.3805, -24.6263) (3.4067, -24.7941) knots 0 0 0 1 2 2 2
  spline S184 degree 2 poles (3.4067, -24.7941) (3.4329, -24.9619) (3.6074, -25.119) (3.7361, -25.1426) knots 0 0 0 1 2 2 2
  spline S185 degree 2 poles (3.7361, -25.1426) (3.8648, -25.1663) (4.2048, -25.1225) (4.336, -25.102) knots 0 0 0 1 2 2 2
  line L229 (4.336, -25.102) -> (4.4977, -25.0768)
  line L230 (4.4977, -25.0768) -> (4.6011, -25.7387)
  line L231 (4.6011, -25.7387) -> (4.4516, -25.7621)
  spline S186 degree 2 poles (4.4516, -25.7621) (4.2808, -25.7888) (3.9958, -25.8646) (3.9023, -25.9261) knots 0 0 0 1 2 2 2
  spline S187 degree 2 poles (3.9023, -25.9261) (3.8092, -25.9906) (3.723, -26.1791) (3.7459, -26.3255) knots 0 0 0 1 2 2 2
  spline S188 degree 2 poles (3.7459, -26.3255) (3.764, -26.4414) (3.8932, -26.5681) (3.9757, -26.5958) knots 0 0 0 1 2 2 2
  spline S189 degree 2 poles (3.9757, -26.5958) (4.0743, -26.6273) (4.3231, -26.6197) (4.4085, -26.6063) knots 0 0 0 1 2 2 2
  spline S190 degree 2 poles (4.4085, -26.6063) (4.5458, -26.5849) (4.8256, -26.4755) (4.9517, -26.4027) knots 0 0 0 1 2 2 2
  spline S191 degree 2 poles (4.9517, -26.4027) (5.0523, -26.3464) (5.2641, -26.182) (5.3138, -26.1399) knots 0 0 0 1 2 2 2
  line L232 (5.3138, -26.1399) -> (5.3931, -26.1275)
  line L233 (5.3931, -26.1275) -> (5.5189, -26.9328)
  spline S192 degree 2 poles (5.5189, -26.9328) (5.3366, -27.0457) (4.702, -27.3042) (4.3573, -27.3581) knots 0 0 0 1 2 2 2
  spline S193 degree 2 poles (4.3573, -27.3581) (4.0217, -27.4105) (3.5094, -27.3718) (3.3179, -27.2861) knots 0 0 0 1 2 2 2
  spline S194 degree 2 poles (3.3179, -27.2861) (3.1071, -27.1972) (2.8577, -26.8611) (2.822, -26.6323) knots 0 0 0 1 2 2 2
  spline S195 degree 2 poles (2.822, -26.6323) (2.7715, -26.309) (3.0683, -25.7689) (3.3624, -25.651) knots 0 0 0 1 2 2 2
  line L234 (3.3624, -25.651) -> (3.3567, -25.6144)
  spline S196 degree 2 poles (3.3567, -25.6144) (3.2196, -25.6171) (2.9481, -25.5595) (2.809, -25.4688) knots 0 0 0 1 2 2 2
  spline S197 degree 2 poles (2.809, -25.4688) (2.6808, -25.3888) (2.4827, -25.101) (2.4494, -24.8874) knots 0 0 0 1 2 2 2
  line L235 (0.756, -23.8048) -> (1.6595, -23.7589)
  line L236 (1.6595, -23.7589) -> (1.7104, -24.7642)
  line L237 (1.7104, -24.7642) -> (0.807, -24.81)
  line L238 (0.807, -24.81) -> (0.756, -23.8048)
  spline S198 degree 2 poles (-2.8448, -25.6018) (-2.8183, -25.1085) (-2.6213, -24.377) (-2.4322, -24.1367) knots 0 0 0 1 2 2 2
  spline S199 degree 2 poles (-2.4322, -24.1367) (-2.2463, -23.8993) (-1.6747, -23.6765) (-1.2739, -23.698) knots 0 0 0 1 2 2 2
  spline S200 degree 2 poles (-1.2739, -23.698) (-0.87, -23.7197) (-0.3286, -24.0023) (-0.1665, -24.2646) knots 0 0 0 1 2 2 2
  spline S201 degree 2 poles (-0.1665, -24.2646) (-0.0041, -24.5237) (0.1137, -25.2659) (0.0872, -25.7592) knots 0 0 0 1 2 2 2
  spline S202 degree 2 poles (0.0872, -25.7592) (0.0601, -26.2648) (-0.1356, -26.9717) (-0.3283, -27.2211) knots 0 0 0 1 2 2 2
  spline S203 degree 2 poles (-0.3283, -27.2211) (-0.5207, -27.4643) (-1.0981, -27.6806) (-1.4866, -27.6598) knots 0 0 0 1 2 2 2
  spline S204 degree 2 poles (-1.4866, -27.6598) (-1.8966, -27.6378) (-2.4315, -27.3493) (-2.5935, -27.084) knots 0 0 0 1 2 2 2
  spline S205 degree 2 poles (-2.5935, -27.084) (-2.7528, -26.825) (-2.8704, -26.0797) (-2.8448, -25.6018) knots 0 0 0 1 2 2 2
  spline S206 degree 2 poles (-1.8859, -25.6533) (-1.9239, -26.3593) (-1.7232, -26.9421) (-1.4489, -26.9568) knots 0 0 0 1 2 2 2
  spline S207 degree 2 poles (-1.4489, -26.9568) (-1.1745, -26.9716) (-0.9095, -26.4138) (-0.8714, -25.7047) knots 0 0 0 1 2 2 2
  spline S208 degree 2 poles (-0.8714, -25.7047) (-0.834, -25.0079) (-1.0372, -24.4157) (-1.3116, -24.401) knots 0 0 0 1 2 2 2
  spline S209 degree 2 poles (-1.3116, -24.401) (-1.5829, -24.3864) (-1.8484, -24.9534) (-1.8859, -25.6533) knots 0 0 0 1 2 2 2
  line L239 (-4.7819, -27.3781) -> (-4.3641, -25.9223)
  line L240 (-4.3641, -25.9223) -> (-3.8475, -26.0149)
  line L241 (-3.8475, -26.0149) -> (-3.9614, -27.5252)
  line L242 (-3.9614, -27.5252) -> (-4.7819, -27.3781)
  line L243 (-5.8426, -27.188) -> (-5.4248, -25.7322)
  line L244 (-5.4248, -25.7322) -> (-4.9081, -25.8248)
  line L245 (-4.9081, -25.8248) -> (-5.022, -27.3351)
  line L246 (-5.022, -27.3351) -> (-5.8426, -27.188)
  line L247 (-11.6695, -25.0988) -> (-9.0672, -22.0234)
  line L248 (-9.0672, -22.0234) -> (-8.1379, -22.3853)
  line L249 (-8.1379, -22.3853) -> (-8.3004, -26.4106)
  line L250 (-8.3004, -26.4106) -> (-9.224, -26.051)
  line L251 (-9.224, -26.051) -> (-9.0603, -23.3415)
  line L252 (-9.0603, -23.3415) -> (-10.769, -25.4494)
  line L253 (-10.769, -25.4494) -> (-11.6695, -25.0988)
  spline S210 degree 2 poles (-15.3521, -20.6847) (-15.0808, -20.2719) (-14.5422, -19.7392) (-14.2578, -19.6268) knots 0 0 0 1 2 2 2
  spline S211 degree 2 poles (-14.2578, -19.6268) (-13.9776, -19.5154) (-13.3716, -19.6108) (-13.0362, -19.8312) knots 0 0 0 1 2 2 2
  spline S212 degree 2 poles (-13.0362, -19.8312) (-12.6982, -20.0534) (-12.3728, -20.5702) (-12.3648, -20.8784) knots 0 0 0 1 2 2 2
  spline S213 degree 2 poles (-12.3648, -20.8784) (-12.3551, -21.1841) (-12.6271, -21.8846) (-12.8984, -22.2974) knots 0 0 0 1 2 2 2
  spline S214 degree 2 poles (-12.8984, -22.2974) (-13.1765, -22.7206) (-13.7016, -23.2327) (-13.9936, -23.3511) knots 0 0 0 1 2 2 2
  spline S215 degree 2 poles (-13.9936, -23.3511) (-14.2823, -23.4643) (-14.8902, -23.3603) (-15.2153, -23.1467) knots 0 0 0 1 2 2 2
  spline S216 degree 2 poles (-15.2153, -23.1467) (-15.5584, -22.9211) (-15.8752, -22.4025) (-15.8816, -22.0917) knots 0 0 0 1 2 2 2
  spline S217 degree 2 poles (-15.8816, -22.0917) (-15.8887, -21.7878) (-15.615, -21.0846) (-15.3521, -20.6847) knots 0 0 0 1 2 2 2
  spline S218 degree 2 poles (-14.5497, -21.2121) (-14.938, -21.803) (-15.0583, -22.4075) (-14.8286, -22.5584) knots 0 0 0 1 2 2 2
  spline S219 degree 2 poles (-14.8286, -22.5584) (-14.599, -22.7093) (-14.0892, -22.3609) (-13.6991, -21.7675) knots 0 0 0 1 2 2 2
  spline S220 degree 2 poles (-13.6991, -21.7675) (-13.3159, -21.1844) (-13.1932, -20.5704) (-13.4228, -20.4195) knots 0 0 0 1 2 2 2
  spline S221 degree 2 poles (-13.4228, -20.4195) (-13.6498, -20.2703) (-14.1647, -20.6264) (-14.5497, -21.2121) knots 0 0 0 1 2 2 2
  spline S222 degree 2 poles (-18.1907, -18.5339) (-17.8706, -18.1699) (-17.1671, -17.7113) (-16.7969, -17.6504) knots 0 0 0 1 2 2 2
  spline S223 degree 2 poles (-16.7969, -17.6504) (-16.4177, -17.5933) (-15.6626, -17.838) (-15.2638, -18.1888) knots 0 0 0 1 2 2 2
  spline S224 degree 2 poles (-15.2638, -18.1888) (-15.1294, -18.307) (-14.8678, -18.5987) (-14.8314, -18.6555) knots 0 0 0 1 2 2 2
  line L254 (-14.8314, -18.6555) -> (-15.3248, -19.2165)
  line L255 (-15.3248, -19.2165) -> (-15.3805, -19.1676)
  spline S225 degree 2 poles (-15.3805, -19.1676) (-15.4093, -19.0929) (-15.5557, -18.8572) (-15.7296, -18.7043) knots 0 0 0 1 2 2 2
  spline S226 degree 2 poles (-15.7296, -18.7043) (-15.871, -18.5799) (-16.1982, -18.4237) (-16.3623, -18.4232) knots 0 0 0 1 2 2 2
  spline S227 degree 2 poles (-16.3623, -18.4232) (-16.5375, -18.4213) (-16.8895, -18.5599) (-17.0799, -18.7296) knots 0 0 0 1 2 2 2
  spline S228 degree 2 poles (-17.0799, -18.7296) (-16.8433, -18.7691) (-16.4893, -18.8995) (-16.2922, -19.0729) knots 0 0 0 1 2 2 2
  spline S229 degree 2 poles (-16.2922, -19.0729) (-16.1462, -19.2013) (-15.9443, -19.5187) (-15.9064, -19.7001) knots 0 0 0 1 2 2 2
  spline S230 degree 2 poles (-15.9064, -19.7001) (-15.8579, -19.9442) (-16.0042, -20.4611) (-16.257, -20.7486) knots 0 0 0 1 2 2 2
  spline S231 degree 2 poles (-16.257, -20.7486) (-16.4548, -20.9735) (-16.9402, -21.2168) (-17.2017, -21.2335) knots 0 0 0 1 2 2 2
  spline S232 degree 2 poles (-17.2017, -21.2335) (-17.4631, -21.2503) (-18.0052, -21.0531) (-18.2532, -20.8349) knots 0 0 0 1 2 2 2
  spline S233 degree 2 poles (-18.2532, -20.8349) (-18.5036, -20.6147) (-18.7684, -20.1351) (-18.7791, -19.8667) knots 0 0 0 1 2 2 2
  spline S234 degree 2 poles (-18.7791, -19.8667) (-18.7986, -19.5617) (-18.5129, -18.9002) (-18.1907, -18.5339) knots 0 0 0 1 2 2 2